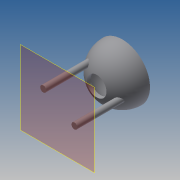
# Autodesk Inventor part: 滑軌
Saved by Autodesk Inventor 2015 (Build 190159000, 159)
## iProperties
Created: 2018-01-06
Part Number: 滑軌
Material: 一般
Document SubType Name: Modeling
Designer: user
Density: 1 g/cm^3
Appearance: 預設
Author: user
Autodesk Inventor part; units mm, degrees
ref_plane "YZ Plane" through (0, 0, 0) normal (1, 0, 0) x (0, 1, 0)
ref_plane "XY Plane" through (0, 0, 0) normal (0, 0, 1) x (1, 0, 0)
sketch "草圖5" plane through (0, 0, 0) normal (0, 0, 1) x (1, 0, 0)
  arc A0 (8, -21.0297) -> (22.5, 0) centre (0, 0) ccw
  line L0 (0, 0) -> (22.5, 0)
  line L1 (0, 0) -> (0, -27.5)
  arc A1 (8, -17.7834) -> (19.5, 0) centre (0, 0) ccw
  line L2 (0, -19.2347) -> (8, -19.2347)
  line L3 (8, -17.7834) -> (8, -21.0297)
  dimension "d12" = 45
  dimension "d13" = 3
  dimension "d14" = 8
  dimension "d20" = 8
  constraints: 8 end point, 4 point on circle, 2 centre point, 2 coincident, 2 horizontal, 2 point on line, 1 perpendicular, 1 vertical
  measures "d12" diameter of A0
  measures "d13" radial gap between concentric circles of A0 A1
  measures "d14" distance from line of L1 L2.end
  measures "d20" distance from line of L3.start L1
revolve "迴轉1" add sketch "草圖5" angle 360 about axis through (0, 0, 0) along (0, -1, 0) contours L3 A1 L0 A0
ref_plane "工作平面1" through (0, -53, 0) normal (0, 1, 0) x (-1, 0, 0)
sketch "草圖6" plane through (0, -53, 0) normal (0, 1, 0) x (-1, 0, 0)
  circle A0 centre (-13.7912, -5.2736) radius 2.4353
  circle A1 centre (11.6639, 8.1939) radius 2.5
  point P0 (0, 0)
  dimension "d19" = 5
  constraints: 2 centre point
  measures "d19" diameter of A1
extrude "擠出2" add sketch "草圖6" along normal up to next
